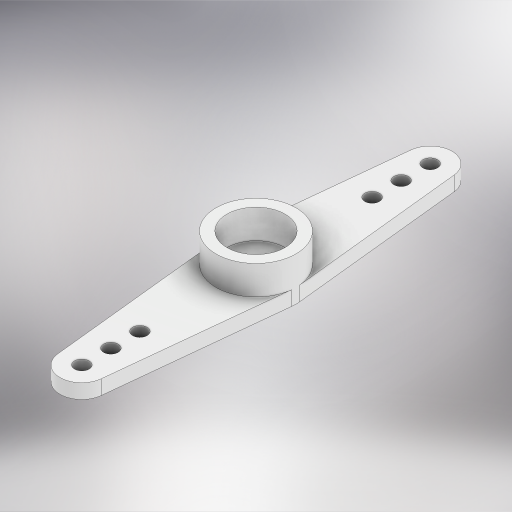
# Autodesk Inventor part: Dual Servo Attachment
Saved by Autodesk Inventor 2024 (Build 280153000, 153)
## iProperties
Created: 2023-04-24
Part Number: Dual Servo Attachment
Material: ABS Plastic
Document SubType Name: Modeling
Designer: byrne
Density: 1.06 g/cm^3
Appearance: Smooth - White
Author: byrne
Autodesk Inventor part; units mm, degrees
ref_plane "YZ Plane" through (0, 0, 0) normal (1, 0, 0) x (0, 1, 0)
ref_plane "XZ Plane" through (0, 0, 0) normal (0, 1, 0) x (-1, 0, 0)
ref_plane "XY Plane" through (0, 0, 0) normal (0, 0, 1) x (1, 0, 0)
sketch "Sketch1" plane through (0, 0, 0) normal (0, 1, 0) x (-1, 0, 0)
  circle A0 centre (0, 0) radius 2.75
  circle A1 centre (0, 12) radius 1.5
  circle A2 centre (0, -12) radius 1.5
  line L0 (0, 12) -> (0, -12) construction
  line L1 (2.735, -0.2865) -> (1.4918, -12.1562)
  line L2 (-1.4918, 12.1563) -> (-2.735, 0.2865)
  line L3 (-1.4918, -12.1562) -> (-2.735, -0.2865)
  line L4 (1.4918, 12.1563) -> (2.735, 0.2865)
  dimension "d0" = 5.5
  dimension "d1" = 3
  dimension "d2" = 27
  constraints: 10 end point, 8 point on circle, 8 tangent, 3 centre point, 2 coincident, 1 equal radius, 1 midpoint, 1 vertical
  measures "d0" diameter of A0
  measures "d1" diameter of A2
extrude "Extrusion1" add sketch "Sketch1" along normal blind 1
sketch "Sketch2" plane through (0, 1, 0) normal (0, 1, 0) x (1, 0, 0)
  circle A0 centre (0, 0) radius 2.75
  circle A1 centre (0, 0) radius 2
  dimension "d5" = 5.5
  dimension "d6" = 4
  constraints: 2 centre point, 2 coincident
  measures "d5" diameter of A0
  measures "d6" diameter of A1
extrude "Extrusion2" add sketch "Sketch2" along normal blind 2
sketch "Sketch3" plane through (0, 0, 0) normal (0, -1, 0) x (1, 0, 0)
  line L0 (-1.4918, -12.1562) -> (-2.735, -0.2865) projected
  arc A0 (-1.4918, -12.1562) -> (1.4918, -12.1562) centre (0, -12) ccw projected
  line L1 (2.735, -0.2865) -> (1.4918, -12.1562) projected
  arc A1 (2.735, -0.2865) -> (2.735, 0.2865) centre (0, 0) ccw projected
  line L2 (1.4918, 12.1563) -> (2.735, 0.2865) projected
  arc A2 (1.4918, 12.1563) -> (-1.4918, 12.1563) centre (0, 12) ccw projected
  line L3 (-2.735, 0.2865) -> (-1.4918, 12.1563) projected
  arc A3 (-2.735, 0.2865) -> (-2.735, -0.2865) centre (0, 0) ccw projected
  circle A4 centre (0, -12) radius 0.5
  circle A5 centre (0, -10) radius 0.5
  circle A6 centre (0, -8) radius 0.5
  circle A7 centre (0, 8) radius 0.5
  circle A8 centre (0, 10) radius 0.5
  circle A9 centre (0, 12) radius 0.5
  dimension "d9" = 1
  dimension "d10" = 1
  dimension "d11" = 1
  dimension "d12" = 1
  dimension "d13" = 1
  dimension "d16" = 180
  constraints: 6 centre point, 2 vertical alignment, 1 coincident, 7 other
  measures "d9" diameter of A4
  measures "d10" diameter of A5
  measures "d11" diameter of A6
extrude "Extrusion3" cut sketch "Sketch3" against normal through all contours A4 | A5 | A6 | A7 | A8 | A9
body "Solid1"
